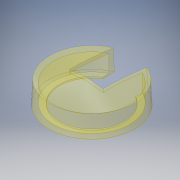
# Autodesk Inventor part: FullTopx
Saved by Autodesk Inventor 2019 (Build 230136000, 136)
## iProperties
Created: 2019-10-06
Part Number: FullTopx
Material: Generic
Document SubType Name: Modeling
Designer: james
Density: 1 g/cm^3
Appearance: Clear - Yellow
Author: james
Autodesk Inventor part; units mm, degrees
ref_plane "YZ Plane" through (0, 0, 0) normal (1, 0, 0) x (0, 1, 0)
ref_plane "XZ Plane" through (0, 0, 0) normal (0, 1, 0) x (-1, 0, 0)
ref_plane "XY Plane" through (0, 0, 0) normal (0, 0, 1) x (1, 0, 0)
sketch "Sketch1" plane through (0, 0, 0) normal (1, 0, 0) x (0, 1, 0)
  line L0 (74.9127, 161.4228) -> (59.7618, 161.4228)
  line L1 (-45.1093, -18.0862) -> (-45.1093, 9.0228)
  line L2 (-45.1093, 9.0228) -> (-51.4593, 9.0228)
  line L3 (-51.4593, 9.0228) -> (-51.4593, -41.7772)
  line L4 (37.2342, -18.0862) -> (-45.1093, -18.0862)
  line L5 (-51.4593, -41.7772) -> (50.0237, -36.9026)
  line L6 (50.0237, -36.9026) -> (74.9127, 161.4228)
  line L7 (59.7618, 161.4228) -> (37.2342, -18.0862)
  point P0 (0, 0)
  dimension "d0" = 101.6
  dimension "d2" = 50.8
  dimension "d3" = 6.35
  dimension "d4" = 87.25
  constraints: 16 end point, 2 perpendicular, 1 horizontal, 1 vertical
  measures "d0" distance of L3.end L5.end
  measures "d2" distance of L2.end L3.end
  measures "d3" distance between parallel lines of L3 L1
  measures "d4" angle of L3 L5
revolve "Revolution1" add sketch "Sketch1" angle 360 about axis through (0, 74.9127, 161.4228) along (0, -1, 0)
sketch "Sketch2" plane through (0, -51.4593, 161.4228) normal (0, -1, 0) x (1, 0, 0)
  line L0 (79.375, 25.4) -> (-79.375, 25.4)
  line L1 (-79.375, 25.4) -> (-79.375, -278.9965)
  line L2 (-79.375, -278.9965) -> (79.375, -278.9965)
  line L3 (79.375, -278.9965) -> (79.375, 25.4)
  circle A0 centre (0, 0) radius 203.2 projected
  point P0 (0, -161.4228)
  dimension "d6" = 158.75
  dimension "d7" = 79.375
  dimension "d8" = 25.4
  constraints: 8 end point, 2 parallel, 1 horizontal, 1 perpendicular
  measures "d6" distance of L1.end L2.end
  measures "d7" distance from line of L3 A0.centre
  measures "d8" distance from line of A0.centre L0
extrude "Extrusion1" cut sketch "Sketch2" against normal blind 127 contours L3 A0 L1 L0 | L3 L2 L1 A0 picked at (-3.0192, -50.7327)
body "Solid1"
